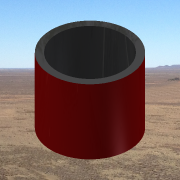
# Autodesk Inventor part: roundNorthBand
Saved by Autodesk Inventor 2014 SP1 (Build 180222100, 222)
## iProperties
Created: 2015-05-21
Part Number: roundNorthBand
Material: Rubber
Document SubType Name: Modeling
Designer: Dave
Mass: 0.33107 g
Surface Area: 11.2274 cm^2
Volume: 0.355989 cm^3
Density: 0.93 g/cm^3
Appearance: Rubber - Black - Version 1.1
Author: Dave
Autodesk Inventor part; units mm, degrees
ref_plane "YZ Plane" through (0, 0, 0) normal (1, 0, 0) x (0, 1, 0)
ref_plane "XZ Plane" through (0, 0, 0) normal (0, 1, 0) x (-1, 0, 0)
ref_plane "XY Plane" through (0, 0, 0) normal (0, 0, 1) x (1, 0, 0)
sketch "Sketch1" plane through (0, 0, 0) normal (0, 1, 0) x (-1, 0, 0)
  circle A0 centre (0, 0) radius 12.7
  circle A1 centre (0, 0) radius 15.24
  dimension "d0" = 25.4
  dimension "d3" = 2.54
  constraints: 2 centre point, 1 coincident
  measures "d0" diameter of A0
  measures "d3" radial gap between concentric circles of A1 A0
extrude "Extrusion1" add sketch "Sketch1" along normal blind 25.4
body "Solid1"
